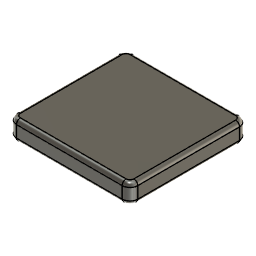
Battery (Autodesk Fusion 360 design; units mm, degrees)
Autodesk Fusion 360 part; units mm, degrees
sketch "Sketch1" plane through (0, 0, 0) normal (0, 0, 1) x (1, 0, 0)
  line L0 (0, 0) -> (31, 0)
  line L1 (31, 0) -> (31, 30)
  line L2 (31, 30) -> (0, 30)
  line L3 (0, 30) -> (0, 0)
  dimension "d1" = 31
  dimension "d2" = 30
  constraint horizontal L0
  constraint vertical L1
  constraint horizontal L2
  constraint vertical L3
  constraint coincident L0.start L3.end
  measures "d1" distance of L0.start L0.end
  measures "d2" distance of L0.start L2.end
extrude "Extrude1" add sketch "Sketch1" along normal blind 5
fillet "Fillet1" radius 2 1 edges at (31, 0, 2.5)
fillet "Fillet2" radius 2 1 edges at (31, 30, 2.5)
fillet "Fillet3" radius 2 1 edges at (0, 30, 2.5)
fillet "Fillet4" radius 2 1 edges at (0, 0, 2.5)
fillet "Fillet5" radius 1 8 edges at (0.5858, 0.5858, 5) (15.5, 0, 5) (30.4142, 0.5858, 5) (31, 15, 5) (30.4142, 29.4142, 5) (15.5, 30, 5) (0.5858, 29.4142, 5) (0, 15, 5)
fillet "Fillet6" radius 1 8 edges at (15.5, 0, 0) (30.4142, 0.5858, 0) (31, 15, 0) (30.4142, 29.4142, 0) (15.5, 30, 0) (0.5858, 29.4142, 0) (0, 15, 0) (0.5858, 0.5858, 0)
